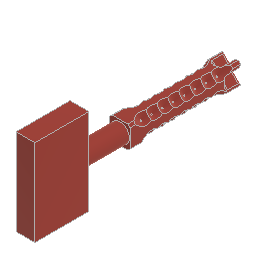
xylok (Autodesk Fusion 360 design; units mm, degrees)
Autodesk Fusion 360 part; units mm, degrees
ref_plane "WorkPlane1" through (0, 22.06, 0) normal (0, 1, 0) x (0, 0, 1)
sketch "rear cross body" plane through (0, 22.06, 0) normal (0, 1, 0) x (1, 0, 0)
  line L0 (0, 0) -> (3.685, 0)
  line L1 (3.685, 0) -> (3.685, -4.12)
  line L2 (3.685, -4.12) -> (0, -4.12)
  line L3 (0, -4.12) -> (0, 0)
  line L4 (0, 0) -> (1.9445, -1.9445) construction
  line L5 (0, 0) -> (3.685, 0) construction
  line L6 (3.685, 0) -> (1.7405, -1.9445) construction
  line L7 (3.685, 0) -> (0, 0) construction
  line L8 (3.685, -4.12) -> (1.7405, -2.1755) construction
  line L9 (3.685, -4.12) -> (0, -4.12) construction
  line L10 (0, -4.12) -> (1.9445, -2.1755) construction
  line L11 (0, -4.12) -> (3.685, -4.12) construction
  line L12 (1.9445, -1.9445) -> (2.3688, -1.5203)
  line L13 (1.9445, -1.9445) -> (1.5203, -2.3688)
  line L14 (1.5203, -2.3688) -> (0, -0.8485)
  line L15 (2.3688, -1.5203) -> (0.8485, 0)
  line L16 (1.7405, -1.9445) -> (1.3162, -1.5203)
  line L17 (1.7405, -1.9445) -> (2.1647, -2.3688)
  line L18 (1.3162, -1.5203) -> (2.8365, 0)
  line L19 (2.1647, -2.3688) -> (3.685, -0.8485)
  line L20 (1.7405, -2.1755) -> (2.1647, -1.7512)
  line L21 (1.7405, -2.1755) -> (1.3162, -2.5997)
  line L22 (2.1647, -1.7512) -> (3.685, -3.2715)
  line L23 (1.3162, -2.5997) -> (2.8365, -4.12)
  line L24 (1.9445, -2.1755) -> (1.5203, -1.7512)
  line L25 (1.9445, -2.1755) -> (2.3688, -2.5997)
  line L26 (1.5203, -1.7512) -> (0, -3.2715)
  line L27 (2.3688, -2.5997) -> (0.8485, -4.12)
  dimension "d5" = 3.685
  dimension "d6" = 4.12
  dimension "d7" = 3.685
  dimension "d8" = 45
  dimension "d9" = 2.75
  dimension "d10" = 45
  dimension "d11" = 2.75
  dimension "d12" = 45
  dimension "d13" = 2.75
  dimension "d14" = 45
  dimension "d15" = 2.75
  dimension "d16" = 0.6
  dimension "d17" = 0.6
  dimension "d18" = 0.6
  dimension "d19" = 0.6
  dimension "d20" = 0.6
  dimension "d21" = 0.6
  dimension "d22" = 0.6
  dimension "d23" = 0.6
  constraint coincident L0.start L3.end
  constraint horizontal L0
  constraint perpendicular L0 L1
  constraint perpendicular L1 L2
  constraint horizontal L5
  constraint horizontal L7
  constraint horizontal L9
  constraint horizontal L11
  constraint perpendicular L4 L12
  constraint perpendicular L4 L13
  constraint coincident L3 L14.end
  constraint perpendicular L13 L14
  constraint coincident L0 L15.end
  constraint perpendicular L12 L15
  constraint perpendicular L6 L16
  constraint perpendicular L6 L17
  constraint coincident L5 L18.end
  constraint perpendicular L4 L18
  constraint coincident L1 L19.end
  constraint perpendicular L17 L19
  constraint perpendicular L8 L20
  constraint perpendicular L8 L21
  constraint coincident L1 L22.end
  constraint perpendicular L20 L22
  constraint coincident L2 L23.end
  constraint perpendicular L10 L23
  constraint perpendicular L10 L24
  constraint perpendicular L10 L25
  constraint coincident L3 L26.end
  constraint perpendicular L24 L26
  constraint coincident L2 L27.end
  constraint perpendicular L8 L27
  measures "d5" distance of L0.start L0.end
  measures "d6" distance of L0.end L1.end
  measures "d7" distance of L1.end L2.end
  measures "d8" angle of L4 L5
  measures "d9" distance of L0.start L4.end
  measures "d10" angle of L6 L7
  measures "d11" distance of L0.end L6.end
  measures "d12" angle of L8 L9
  measures "d13" distance of L1.end L8.end
  measures "d14" angle of L10 L11
  measures "d15" distance of L2.end L10.end
  measures "d16" distance of L4.end L12.end
  measures "d17" distance of L4.end L13.end
  measures "d18" distance of L6.end L16.end
  measures "d19" distance of L6.end L17.end
  measures "d20" distance of L8.end L20.end
  measures "d21" distance of L8.end L21.end
  measures "d22" distance of L10.end L24.end
  measures "d23" distance of L10.end L25.end
extrude "Extrude1" add sketch "rear cross body" against normal blind 1.51 contours L0 L3 L13 L14 L15 L16 L17 L18 L24 L26 | L0 L1 L12 L13 L15 L17 L18 L19 L20 L22 | L12 L13 L15 L16 L17 L18 | L2 L3 L13 L14 L20 L21 L23 L24 L26 L27 | L13 L14 L24 L26 | L13 L17 L20 L24 | L1 L2 L17 L19 L20 L22 L23 L24 L25 L27 | L17 L19 L20 L22 | L20 L21 L23 L24 L25 L27 makes body 1
sketch "core" plane through (0, 0, 0) normal (0, 1, 0) x (1, 0, 0)
  line L0 (0, 0) -> (1.8425, 0) construction
  line L1 (1.8425, 0) -> (1.8425, -2.06) construction
  circle A0 centre (1.8425, -2.06) radius 2.525
  circle A1 centre (1.8425, -2.06) radius 5.75
  dimension "d26" = 1.8425
  dimension "d27" = 2.06
  dimension "d28" = 5.05
  dimension "d29" = 11.5
  constraint coincident L0.start origin
  constraint horizontal L0
  constraint perpendicular L0 L1
  constraint coincident L1.end A0.centre
  constraint concentric A0 A1
  measures "d26" distance of L0.start L0.end
  measures "d27" distance of L0.end L1.end
  measures "d28" diameter of A0
  measures "d29" diameter of A1
extrude "Extrude2" add sketch "core" along normal blind 22.06 separate body makes body 2
move_body "Move1" bodies 1 to x (0.707107, 0, -0.707107) y (0, 1, 0) z (0.707107, 0, 0.707107) at (-0.917, 0, 1.9062)
sketch "rear cross negative" plane through (0, 22.06, 0) normal (0, 1, 0) x (-1, 0, 0)
  circle A0 centre (-1.8425, 2.06) radius 2.525
  circle A1 centre (-1.8425, 2.06) radius 5.75
  line L0 (0, 0) -> (-1.8425, 0) construction
  line L1 (-1.8425, 0) -> (-1.8425, 2.06) construction
  line L2 (-1.8425, 2.06) -> (-1.3786, 2.5239) construction
  line L3 (-1.8425, 2.06) -> (-1.1865, 2.06) construction
  line L4 (-1.8425, 2.06) -> (-1.071, 1.2885) construction
  line L5 (-1.8425, 2.06) -> (-0.7515, 2.06) construction
  line L6 (-1.8425, 2.06) -> (-2.3064, 1.5961) construction
  line L7 (-1.8425, 2.06) -> (-2.4985, 2.06) construction
  line L8 (-1.8425, 2.06) -> (-2.614, 2.8315) construction
  line L9 (-1.8425, 2.06) -> (-2.9335, 2.06) construction
  line L10 (-1.3786, 2.5239) -> (-1.3786, 4.542)
  line L11 (-1.3786, 2.5239) -> (0.6395, 2.5239)
  line L12 (-1.071, 1.2885) -> (0.5618, 1.2885)
  line L13 (-1.071, 1.2885) -> (-1.071, -0.3443)
  line L14 (-2.3064, 1.5961) -> (-2.3064, -0.422)
  line L15 (-2.3064, 1.5961) -> (-4.3245, 1.5961)
  line L16 (-2.614, 2.8315) -> (-4.2468, 2.8315)
  line L17 (-2.614, 2.8315) -> (-2.614, 4.4643)
  circle A2 centre (-1.8425, 2.06) radius 1
  point P0 (-1.3963, 2.5062)
  point P1 (-1.0887, 1.3062)
  dimension "d33" = 1.8425
  dimension "d34" = 2.06
  dimension "d35" = 0.4462
  dimension "d36" = 0.4462
  dimension "d37" = 0.7538
  dimension "d38" = 0.7538
  dimension "d39" = 45
  dimension "d40" = 0.656
  dimension "d41" = 45
  dimension "d42" = 1.091
  dimension "d43" = 45
  dimension "d44" = 0.656
  dimension "d45" = 45
  dimension "d46" = 1.091
  dimension "d47" = 2
  constraint coincident L0.start origin
  constraint horizontal L0
  constraint perpendicular L0 L1
  constraint horizontal L3
  constraint horizontal L5
  constraint coincident A0.centre A1.centre
  constraint horizontal L7
  constraint horizontal L9
  constraint coincident A0 L10.end
  constraint perpendicular L9 L10
  constraint coincident A0 L11.end
  constraint perpendicular L10 L11
  constraint coincident A0 L12.end
  constraint parallel L11 L12
  constraint coincident A0 L13.end
  constraint perpendicular L0 L13
  constraint coincident A0 L14.end
  constraint parallel L1 L14
  constraint coincident A0 L15.end
  constraint perpendicular L14 L15
  constraint coincident A0 L16.end
  constraint parallel L15 L16
  constraint coincident A0 L17.end
  constraint perpendicular L16 L17
  measures "d33" distance of L0.start L0.end
  measures "d34" distance of L0.end A0.centre
  measures "d35" horizontal distance of A0.centre P0
  measures "d36" vertical distance of A0.centre P0
  measures "d37" horizontal distance of A0.centre P1
  measures "d38" vertical distance of A0.centre P1
  measures "d39" angle of L2 L3
  measures "d40" distance of A0.centre L2.end
  measures "d41" angle of L4 L5
  measures "d42" distance of A0.centre L4.end
  measures "d43" angle of L6 L7
  measures "d44" distance of A0.centre L6.end
  measures "d45" angle of L8 L9
  measures "d46" distance of A0.centre L8.end
  measures "d47" diameter of A2
extrude "Extrude3" add sketch "rear cross negative" against normal blind 1.51 contours A0 L10 L11 A2 | A0 L12 L13 | A0 L16 L17 | A0 L14 L15 A2 bodies 2
ref_plane "WorkPlane2" through (1.8425, 8.7609, 7.81) normal (0, 0, 1) x (-1, 0, 0)
ref_plane "WorkPlane3" through (7.5925, 14.4539, 2.06) normal (1, 0, 0) x (0, 0, 1)
ref_plane "WorkPlane4" through (-3.9075, 8.1447, 2.06) normal (-1, 0, 0) x (0, 0, -1)
ref_plane "WorkPlane5" through (1.8425, 3.131, -3.69) normal (0, 0, -1) x (1, 0, 0)
sketch "top" plane through (0, 0, 7.81) normal (0, 0, 1) x (1, 0, 0)
  line L0 (0, 0) -> (1.8425, 0) construction
  line L1 (1.8425, 0) -> (1.8425, 4.2) construction
  line L2 (1.8425, 4.2) -> (1.8425, 5.68) construction
  circle A0 centre (1.8425, 5.68) radius 1.48
  line L3 (1.8425, 5.68) -> (1.8425, 9.7) construction
  circle A1 centre (1.8425, 9.7) radius 1.48
  line L4 (1.8425, 9.7) -> (1.8425, 13.72) construction
  circle A2 centre (1.8425, 13.72) radius 1.48
  line L5 (1.8425, 13.72) -> (1.8425, 17.74) construction
  circle A3 centre (1.8425, 17.74) radius 1.48
  dimension "d54" = 1.8425
  dimension "d55" = 4.2
  dimension "d56" = 1.48
  dimension "d57" = 2.96
  dimension "d58" = 4.02
  dimension "d59" = 2.96
  dimension "d60" = 4.02
  dimension "d61" = 2.96
  dimension "d62" = 4.02
  dimension "d63" = 2.96
  constraint coincident L0.start origin
  constraint horizontal L0
  constraint perpendicular L0 L1
  constraint parallel L1 L2
  constraint coincident L2.end A0.centre
  constraint parallel L2 L3
  constraint coincident L3.end A1.centre
  constraint parallel L3 L4
  constraint coincident L4.end A2.centre
  constraint parallel L4 L5
  constraint coincident L5.end A3.centre
  measures "d54" distance of L0.start L0.end
  measures "d55" distance of L0.end L1.end
  measures "d56" distance of L1.end L2.end
  measures "d57" diameter of A0
  measures "d58" distance of L2.end L3.end
  measures "d59" diameter of A1
  measures "d60" distance of L3.end L4.end
  measures "d61" diameter of A2
  measures "d62" distance of L4.end L5.end
  measures "d63" diameter of A3
sketch "right" plane through (7.5925, 0, 0) normal (1, 0, 0) x (0, 1, 0)
  line L0 (0, 0) -> (0, 2.06) construction
  line L1 (0, 2.06) -> (5.1, 2.06) construction
  line L2 (5.1, 2.06) -> (6.58, 2.06) construction
  circle A0 centre (6.58, 2.06) radius 1.48
  line L3 (6.58, 2.06) -> (10.6, 2.06) construction
  circle A1 centre (10.6, 2.06) radius 1.48
  line L4 (10.6, 2.06) -> (14.62, 2.06) construction
  circle A2 centre (14.62, 2.06) radius 1.48
  line L5 (14.62, 2.06) -> (18.64, 2.06) construction
  circle A3 centre (18.64, 2.06) radius 1.48
  dimension "d64" = 2.06
  dimension "d65" = 5.1
  dimension "d66" = 1.48
  dimension "d67" = 2.96
  dimension "d68" = 4.02
  dimension "d69" = 2.96
  dimension "d70" = 4.02
  dimension "d71" = 2.96
  dimension "d72" = 4.02
  dimension "d73" = 2.96
  constraint coincident L0.start origin
  constraint vertical L0
  constraint perpendicular L0 L1
  constraint parallel L1 L2
  constraint coincident L2.end A0.centre
  constraint parallel L2 L3
  constraint coincident L3.end A1.centre
  constraint parallel L3 L4
  constraint coincident L4.end A2.centre
  constraint parallel L4 L5
  constraint coincident L5.end A3.centre
  measures "d64" distance of L0.start L0.end
  measures "d65" distance of L0.end L1.end
  measures "d66" distance of L1.end L2.end
  measures "d67" diameter of A0
  measures "d68" distance of L2.end L3.end
  measures "d69" diameter of A1
  measures "d70" distance of L3.end L4.end
  measures "d71" diameter of A2
  measures "d72" distance of L4.end L5.end
  measures "d73" diameter of A3
sketch "bottom" plane through (0, 0, -3.69) normal (0, 0, -1) x (-1, 0, 0)
  line L0 (0, 0) -> (-1.8425, 0) construction
  line L1 (-1.8425, 0) -> (-1.8425, 6.2) construction
  line L2 (-1.8425, 6.2) -> (-1.8425, 7.68) construction
  circle A0 centre (-1.8425, 7.68) radius 1.48
  line L3 (-1.8425, 7.68) -> (-1.8425, 11.7) construction
  circle A1 centre (-1.8425, 11.7) radius 1.48
  line L4 (-1.8425, 11.7) -> (-1.8425, 15.72) construction
  circle A2 centre (-1.8425, 15.72) radius 1.48
  dimension "d74" = 1.8425
  dimension "d75" = 6.2
  dimension "d76" = 1.48
  dimension "d77" = 2.96
  dimension "d78" = 4.02
  dimension "d79" = 2.96
  dimension "d80" = 4.02
  dimension "d81" = 2.96
  constraint coincident L0.start origin
  constraint horizontal L0
  constraint perpendicular L0 L1
  constraint parallel L1 L2
  constraint coincident L2.end A0.centre
  constraint parallel L2 L3
  constraint coincident L3.end A1.centre
  constraint parallel L3 L4
  constraint coincident L4.end A2.centre
  measures "d74" distance of L0.start L0.end
  measures "d75" distance of L0.end L1.end
  measures "d76" distance of L1.end L2.end
  measures "d77" diameter of A0
  measures "d78" distance of L2.end L3.end
  measures "d79" diameter of A1
  measures "d80" distance of L3.end L4.end
  measures "d81" diameter of A2
sketch "left" plane through (-3.9075, 0, 0) normal (-1, 0, 0) x (0, -1, 0)
  line L0 (0, 0) -> (0, 2.06) construction
  line L1 (0, 2.06) -> (-3.1, 2.06) construction
  line L2 (-3.1, 2.06) -> (-4.58, 2.06) construction
  circle A0 centre (-4.58, 2.06) radius 1.48
  line L3 (-4.58, 2.06) -> (-8.6, 2.06) construction
  circle A1 centre (-8.6, 2.06) radius 1.48
  line L4 (-8.6, 2.06) -> (-12.62, 2.06) construction
  circle A2 centre (-12.62, 2.06) radius 1.48
  line L5 (-12.62, 2.06) -> (-16.64, 2.06) construction
  circle A3 centre (-16.64, 2.06) radius 1.48
  dimension "d82" = 2.06
  dimension "d83" = 3.1
  dimension "d84" = 1.48
  dimension "d85" = 2.96
  dimension "d86" = 4.02
  dimension "d87" = 2.96
  dimension "d88" = 4.02
  dimension "d89" = 2.96
  dimension "d90" = 4.02
  dimension "d91" = 2.96
  constraint coincident L0.start origin
  constraint vertical L0
  constraint perpendicular L0 L1
  constraint parallel L1 L2
  constraint coincident L2.end A0.centre
  constraint parallel L2 L3
  constraint coincident L3.end A1.centre
  constraint parallel L3 L4
  constraint coincident L4.end A2.centre
  constraint parallel L4 L5
  constraint coincident L5.end A3.centre
  measures "d82" distance of L0.start L0.end
  measures "d83" distance of L0.end L1.end
  measures "d84" distance of L1.end L2.end
  measures "d85" diameter of A0
  measures "d86" distance of L2.end L3.end
  measures "d87" diameter of A1
  measures "d88" distance of L3.end L4.end
  measures "d89" diameter of A2
  measures "d90" distance of L4.end L5.end
  measures "d91" diameter of A3
extrude "Extrude4" cut sketch "top" against normal blind 4 bodies 2
extrude "Extrude5" cut sketch "right" against normal blind 4 bodies 2
extrude "Extrude6" cut sketch "bottom" against normal blind 4 bodies 2
extrude "Extrude7" cut sketch "left" against normal blind 4 bodies 2
sketch "key profile" plane through (0, 0, 0) normal (0, 1, 0) x (1, 0, 0)
  line L0 (0, 0) -> (3.685, 0)
  line L1 (3.685, 0) -> (3.685, -4.12)
  line L2 (3.685, -4.12) -> (0, -4.12)
  line L3 (0, -4.12) -> (0, 0)
  dimension "d105" = 3.685
  dimension "d106" = 4.12
  dimension "d107" = 3.685
  constraint coincident L0.start L3.end
  constraint horizontal L0
  constraint perpendicular L0 L1
  constraint perpendicular L1 L2
  measures "d105" distance of L0.start L0.end
  measures "d106" distance of L0.end L1.end
  measures "d107" distance of L1.end L2.end
extrude "Extrude8" add sketch "key profile" along normal blind 20.45 from surface at 1.61 separate body makes body 3
move_face "OffsetFaces4" offset 0.03 2 faces at (3.685, 8.4267, 1.3733) (0, 8.4267, 2.7467) on bodies 3
move_face "OffsetFaces5" offset 0.025 2 faces at (2.4667, 8.4267, 4.12) (1.2183, 8.4267, 0) on bodies 3
move_body "Move2" bodies 3 to x (0.707107, 0, -0.707107) y (0, 1, 0) z (0.707107, 0, 0.707107) at (-0.917, 0, 1.9062)
extrude "Extrude9" cut sketch "core" along normal blind 23 bodies 3
combine "Combine1" operation cut target body 3 tool bodies 2 keep tools
move_face "OffsetFaces1" offset -0.4 2 faces at (0.9761, 21.5567, 2.5593) (2.7089, 21.5567, 1.5607) on bodies 3
move_face "OffsetFaces2" offset -1.49 4 faces at (3.0825, 20.55, 3.3) (0.8052, 20.55, 3.0973) (0.6025, 20.55, 0.82) (2.8798, 20.55, 1.0227) on bodies 3
fillet "Fillet1" radius 0.45 8 edges at (2.614, 22.06, 3.5343) (1.3786, 22.06, 3.3841) (0.5184, 22.06, 2.5239) (0.3682, 22.06, 1.2885) (1.071, 22.06, 0.5857) (2.3064, 22.06, 0.7359) (3.1666, 22.06, 1.5961) (3.3168, 22.06, 2.8315) on bodies 3
move_face "OffsetFaces3" [suppressed]
fillet "Fillet2" radius 0.6 8 edges at (2.614, 19.06, 3.5343) (3.3168, 19.06, 2.8315) (1.3786, 19.06, 3.3841) (0.5184, 19.06, 2.5239) (0.3682, 19.06, 1.2885) (1.071, 19.06, 0.5857) (2.3064, 19.06, 0.7359) (3.1666, 19.06, 1.5961) on bodies 3
extrude "Extrude10" add sketch "top" against normal blind 4.23 from surface at -0.3 separate body contours A0 makes body 4
extrude "Extrude11" add sketch "top" against normal blind 4.23 from surface at -0.3 separate body contours A1 makes body 5
extrude "Extrude12" add sketch "top" against normal blind 4.23 from surface at -0.3 separate body contours A2 makes body 6
extrude "Extrude13" add sketch "top" against normal blind 4.23 from surface at -0.3 separate body contours A3 makes body 7
extrude "Extrude14" add sketch "right" against normal blind 4.23 from surface at -0.3 separate body contours A0 makes body 8
extrude "Extrude15" add sketch "right" against normal blind 4.23 from surface at -0.3 separate body contours A1 makes body 9
extrude "Extrude16" add sketch "right" against normal blind 4.23 from surface at -0.3 separate body contours A2 makes body 10
extrude "Extrude17" add sketch "right" against normal blind 4.23 from surface at -0.3 separate body contours A3 makes body 11
extrude "Extrude18" add sketch "bottom" against normal blind 4.23 from surface at -0.3 separate body contours A0 makes body 12
extrude "Extrude19" add sketch "bottom" against normal blind 4.23 from surface at -0.3 separate body contours A1 makes body 13
extrude "Extrude20" add sketch "bottom" against normal blind 4.23 from surface at -0.3 separate body contours A2 makes body 14
extrude "Extrude21" add sketch "left" against normal blind 4.23 from surface at -0.3 separate body contours A0 makes body 15
extrude "Extrude22" add sketch "left" against normal blind 4.23 from surface at -0.3 separate body contours A1 makes body 16
extrude "Extrude23" add sketch "left" against normal blind 4.23 from surface at -0.3 separate body contours A2 makes body 17
extrude "Extrude24" add sketch "left" against normal blind 4.23 from surface at -0.3 separate body contours A3 makes body 18
chamfer "Chamfer1" distance 1.37 angle 45 15 edges at (0.6225, 5.9598, 2.5952) (0.6225, 9.9798, 2.5952) (3.2223, 8.2152, 0.84) (0.4627, 14.2552, 3.28) (3.2223, 12.2352, 0.84) (3.0625, 9.2202, 2.5952) (3.2223, 16.2552, 0.84) (0.6225, 18.0198, 2.5952) (0.4627, 6.2152, 3.28) (3.0625, 5.2002, 2.5952) (0.6225, 13.9998, 2.5952) (3.0625, 17.2602, 2.5952) (0.4627, 18.2752, 3.28) (3.0625, 13.2402, 2.5952) (0.4627, 10.2352, 3.28) on bodies 4 5 6 7 8 9 10 11 12 13 14 15 16 17 18
extrude "Extrude25" add 1 faces at (1.8708, 5.7087, 3.28) along direction (0, 0, 1) blind 1.37 draft 55 on bodies 4 bodies 4
extrude "Extrude26" add 1 faces at (1.8792, 9.6501, 3.28) along direction (0, 0, 1) blind 1.37 draft 55 on bodies 5 bodies 5
extrude "Extrude27" add 1 faces at (1.8792, 13.6701, 3.28) along direction (0, 0, 1) blind 1.37 draft 55 on bodies 6 bodies 6
extrude "Extrude28" add 1 faces at (1.8728, 17.7193, 3.28) along direction (0, 0, 1) blind 1.37 draft 55 on bodies 7 bodies 7
extrude "Extrude32" add 1 faces at (3.0625, 6.6069, 2.0436) along direction (1, 0, 0) blind 1.37 draft 55 on bodies 8 bodies 8
extrude "Extrude31" add 1 faces at (3.0625, 10.5771, 1.9995) along direction (1, 0, 0) blind 1.37 draft 55 on bodies 9 bodies 9 10
extrude "Extrude30" add 1 faces at (3.0625, 14.5971, 1.9995) along direction (1, 0, 0) blind 1.37 draft 55 on bodies 10 bodies 10
extrude "Extrude29" add 1 faces at (3.0625, 18.6669, 2.0849) along direction (1, 0, 0) blind 1.37 draft 55 on bodies 11 bodies 11
extrude "Extrude33" add 1 faces at (1.8457, 7.7134, 0.84) along direction (0, 0, -1) blind 1.37 draft 55 on bodies 12 bodies 12
extrude "Extrude34" add 1 faces at (1.8058, 11.6682, 0.84) along direction (0, 0, -1) blind 1.37 draft 55 on bodies 13 bodies 13
extrude "Extrude35" add 1 faces at (1.8062, 15.6936, 0.84) along direction (0, 0, -1) blind 1.37 draft 55 on bodies 14 bodies 14
extrude "Extrude36" add 1 faces at (0.6225, 4.5335, 2.0349) along direction (-1, 0, 0) blind 1.37 draft 55 on bodies 15 bodies 15
extrude "Extrude37" add 1 faces at (0.6225, 8.5731, 2.0959) along direction (-1, 0, 0) blind 1.37 draft 55 on bodies 16 bodies 16
extrude "Extrude38" add 1 faces at (0.6225, 12.5931, 2.0959) along direction (-1, 0, 0) blind 1.37 draft 55 on bodies 17 bodies 17
extrude "Extrude39" add 1 faces at (0.6225, 16.6763, 2.0655) along direction (-1, 0, 0) blind 1.37 draft 55 on bodies 18 bodies 18
combine "Combine3" operation cut target body 3 tool bodies 4 5 6 7 8 9 10 11 12 13 14 15 16 17 18 keep tools
move_body "Move4" bodies 3 to x (-1, 0, 0) y (0, 1, 0) z (0, 0, -1) at (3.685, 0, 4.12)
combine "Combine4" operation cut target body 3 tool bodies 4 5 6 7 8 9 10 11 12 13 14 15 16 17 18 keep tools
move_body "Move5" bodies 3 to x (0.707107, 0, 0.707107) y (0, 1, 0) z (-0.707107, 0, 0.707107) at (1.9963, 0, -0.6995)
sketch "bow shaft" plane through (0, 1.61, 0) normal (0, -1, 0) x (1, 0, 0)
  arc A0 (3.715, 3.7539) -> (3.2667, 4.145) centre (1.8425, 2.06) ccw
  line L0 (3.2667, 4.145) -> (0.4183, 4.145)
  arc A1 (0.4183, 4.145) -> (-0.03, 3.7539) centre (1.8425, 2.06) ccw
  line L1 (-0.03, 3.7539) -> (-0.03, 0.3661)
  arc A2 (-0.03, 0.3661) -> (0.4183, -0.025) centre (1.8425, 2.06) ccw
  line L2 (0.4183, -0.025) -> (3.2667, -0.025)
  arc A3 (3.2667, -0.025) -> (3.715, 0.3661) centre (1.8425, 2.06) ccw
  line L3 (3.715, 0.3661) -> (3.715, 3.7539)
  circle A4 centre (1.8425, 2.06) radius 1.75
  dimension "d215" = 3.5
  constraint concentric A0 A4
  measures "d215" diameter of A4
extrude "Extrude40" add sketch "bow shaft" along normal blind 7.5 contours A4 bodies 3
sketch "bow head" plane through (0, -5.89, 0) normal (0, -1, 0) x (1, 0, 0)
  circle A0 centre (1.8425, 2.06) radius 1.75
  line L0 (1.8425, 2.06) -> (0.0925, 2.06) construction
  line L1 (0.0925, 2.06) -> (0.0925, 10.06)
  line L2 (0.0925, 10.06) -> (3.5925, 10.06)
  line L3 (3.5925, 10.06) -> (3.5925, -5.94)
  line L4 (3.5925, -5.94) -> (0.0925, -5.94)
  line L5 (0.0925, -5.94) -> (0.0925, 2.06)
  dimension "d218" = 8
  dimension "d219" = 3.5
  dimension "d220" = 16
  dimension "d221" = 3.5
  constraint coincident A0.centre L0.start
  constraint coincident A0 L0.end
  constraint horizontal L0
  constraint perpendicular L0 L1
  constraint perpendicular L1 L2
  constraint perpendicular L2 L3
  constraint perpendicular L3 L4
  measures "d218" distance of L0.end L1.end
  measures "d219" distance of L1.end L2.end
  measures "d220" distance of L2.end L3.end
  measures "d221" distance of L3.end L4.end
extrude "Extrude41" add sketch "bow head" along normal blind 10 bodies 3
hidden bodies 1 2
equation "pin_extrude_offset = -0.3 mm"
equation "tension_cross_tolerance = 0.025 mm"
equation "ramp_deg = 55 deg"
equation "d7 = d5"
equation "d10 = d8"
equation "d11 = d9"
equation "d12 = d8"
equation "d13 = d9"
equation "d14 = d8"
equation "d15 = d9"
equation "d17 = d16"
equation "d18 = d16"
equation "d19 = d16"
equation "d20 = d16"
equation "d21 = d16"
equation "d22 = d16"
equation "d23 = d16"
equation "d24 = -( 22.06 mm - 20.55 mm )"
equation "d26 = 0.5 * d5"
equation "d27 = 0.5 * d6"
equation "d33 = 0.5 * d5"
equation "d34 = 0.5 * d6"
equation "d40 = sqrt(( ( d35 ^ 2 ) ) + ( ( d36 ^ 2 ) )) + tension_cross_tolerance"
equation "d41 = d39"
equation "d42 = sqrt(( ( d37 ^ 2 ) ) + ( ( d38 ^ 2 ) )) + tension_cross_tolerance"
equation "d43 = d39"
equation "d44 = d40"
equation "d45 = d39"
equation "d46 = d42"
equation "d54 = 0.5 * d5"
equation "d56 = ( 2.96 * 0.5 ) * 1 mm"
equation "d58 = 1.06 mm + d56 * 2"
equation "d59 = d57"
equation "d60 = d58"
equation "d61 = d57"
equation "d62 = d58"
equation "d63 = d57"
equation "d64 = 0.5 * d6"
equation "d66 = d56"
equation "d67 = d57"
equation "d68 = d58"
equation "d69 = d57"
equation "d70 = d58"
equation "d71 = d57"
equation "d72 = d58"
equation "d73 = d57"
equation "d74 = 0.5 * d5"
equation "d76 = d56"
equation "d77 = d57"
equation "d78 = d58"
equation "d79 = d57"
equation "d80 = d58"
equation "d81 = d57"
equation "d82 = 0.5 * d6"
equation "d84 = d56"
equation "d85 = d57"
equation "d86 = d58"
equation "d87 = d57"
equation "d88 = d58"
equation "d89 = d57"
equation "d90 = d58"
equation "d91 = d57"
equation "d92 = -4.00 mm"
equation "d94 = d92"
equation "d96 = d92"
equation "d98 = d92"
equation "max_lift = -3.24 mm"
equation "mid_lift = -3.72 mm"
equation "min_lift = -4.23 mm"
equation "no_pin = -2.5 mm"
equation "pin_ramp_extrude = -1.37 mm"
equation "d105 = d5"
equation "d106 = d6"
equation "d107 = d5"
equation "d109 = 22.06 mm - 1.61 mm"
equation "d116 = -0.25 mm - 1.24 mm"
equation "t1 = min_lift"
equation "t2 = min_lift"
equation "t3 = min_lift"
equation "t4 = min_lift"
equation "r1 = min_lift"
equation "r2 = min_lift"
equation "r3 = min_lift"
equation "r4 = min_lift"
equation "b1 = min_lift"
equation "b2 = min_lift"
equation "b3 = min_lift"
equation "l1 = min_lift"
equation "l2 = min_lift"
equation "l3 = min_lift"
equation "l4 = min_lift"
equation "d137 = pin_extrude_offset"
equation "d138 = t1"
equation "d140 = pin_extrude_offset"
equation "d141 = t2"
equation "d143 = pin_extrude_offset"
equation "d144 = t3"
equation "d146 = pin_extrude_offset"
equation "d147 = t4"
equation "d149 = pin_extrude_offset"
equation "d150 = r1"
equation "d152 = pin_extrude_offset"
equation "d153 = r2"
equation "d155 = pin_extrude_offset"
equation "d156 = r3"
equation "d158 = pin_extrude_offset"
equation "d159 = r4"
equation "d161 = pin_extrude_offset"
equation "d162 = b1"
equation "d164 = pin_extrude_offset"
equation "d165 = b2"
equation "d167 = pin_extrude_offset"
equation "d168 = b3"
equation "d170 = pin_extrude_offset"
equation "d171 = l1"
equation "d173 = pin_extrude_offset"
equation "d174 = l2"
equation "d176 = pin_extrude_offset"
equation "d177 = l3"
equation "d179 = pin_extrude_offset"
equation "d180 = l4"
equation "d182 = -pin_ramp_extrude"
equation "d183 = pin_ramp_extrude"
equation "d184 = ramp_deg"
equation "d185 = pin_ramp_extrude"
equation "d186 = ramp_deg"
equation "d187 = pin_ramp_extrude"
equation "d188 = ramp_deg"
equation "d189 = pin_ramp_extrude"
equation "d190 = ramp_deg"
equation "d191 = pin_ramp_extrude"
equation "d192 = ramp_deg"
equation "d193 = pin_ramp_extrude"
equation "d194 = ramp_deg"
equation "d195 = pin_ramp_extrude"
equation "d196 = ramp_deg"
equation "d197 = pin_ramp_extrude"
equation "d198 = ramp_deg"
equation "d199 = pin_ramp_extrude"
equation "d200 = ramp_deg"
equation "d201 = pin_ramp_extrude"
equation "d202 = ramp_deg"
equation "d203 = pin_ramp_extrude"
equation "d204 = ramp_deg"
equation "d205 = pin_ramp_extrude"
equation "d206 = ramp_deg"
equation "d207 = pin_ramp_extrude"
equation "d208 = ramp_deg"
equation "d209 = pin_ramp_extrude"
equation "d210 = ramp_deg"
equation "d211 = pin_ramp_extrude"
equation "d212 = ramp_deg"
equation "d220 = d218 * 2"
equation "d221 = d219"
named bodies: "rear cross", "core", "key", "t1", "t2", "t3", "t4", "r1", "r2", "r3", "r4", "b1", "b2", "b3", "l1", "l2", "l3", "l4"
